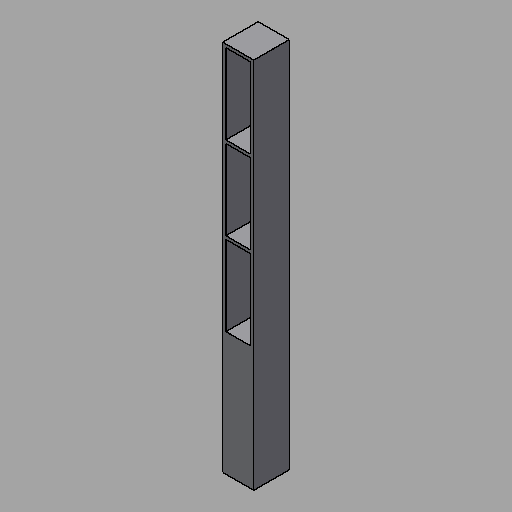
# Autodesk Inventor part: Mobiletto verticale
Saved by Autodesk Inventor 2025.2 (Build 292293000, 293)
## iProperties
Created: 2025-09-19
Part Number: Mobiletto verticale
Material: Generico
Document SubType Name: Modeling
Designer: Limonta
Mass: 39347.7 g
Surface Area: 22881.9 cm^2
Volume: 39347.7 cm^3
Density: 1 g/cm^3
Appearance: Default
FORNITO DA: SBE
Author: Limonta
Autodesk Inventor part; units mm, degrees
ref_plane "YZ Plane" through (0, 0, 0) normal (1, 0, 0) x (0, 1, 0)
ref_plane "XZ Plane" through (0, 0, 0) normal (0, 1, 0) x (-1, 0, 0)
ref_plane "XY Plane" through (0, 0, 0) normal (0, 0, 1) x (1, 0, 0)
sketch "Schizzo1" plane through (0, 0, 0) normal (0, 0, 1) x (1, 0, 0)
  line L0 (-87.5, 0) -> (87.5, 0)
  line L1 (87.5, 0) -> (87.5, 2100)
  line L2 (87.5, 2100) -> (-87.5, 2100)
  line L3 (-87.5, 2100) -> (-87.5, 0)
  point P0 (0, 0)
  point P1 (0, 0)
  dimension "d0" = 175
  dimension "d1" = 2100
  constraints: 8 end point, 2 parallel, 1 coincident, 1 horizontal, 1 midpoint, 1 perpendicular
  measures "d0" distance of L0.start L0.end
  measures "d1" distance of L2.end L0.start
extrude "Estrusione1" add sketch "Schizzo1" against normal blind 200
shell "Svuotamento1" thickness 18 removed faces 1 at (-29.1667, 1400, 0)
sketch "Schizzo2" plane through (0, 0, 0) normal (0, 0, 1) x (1, 0, 0)
  line L0 (-69.5, 18) -> (-69.5, 2082) projected
  line L1 (69.5, 2082) -> (69.5, 18) projected
  line L2 (-69.5, 1632) -> (69.5, 1632)
  line L3 (69.5, 1632) -> (69.5, 1614)
  line L4 (69.5, 1614) -> (-69.5, 1614)
  line L5 (-69.5, 1614) -> (-69.5, 1632)
  line L6 (-69.5, 1164) -> (69.5, 1164)
  line L7 (69.5, 1164) -> (69.5, 1146)
  line L8 (69.5, 1146) -> (-69.5, 1146)
  line L9 (-69.5, 1146) -> (-69.5, 1164)
  line L10 (-69.5, 18) -> (-69.5, 2082) projected
  line L11 (69.5, 2082) -> (69.5, 18) projected
  line L12 (-69.5, 696) -> (69.5, 696)
  line L13 (69.5, 696) -> (69.5, 18)
  line L14 (69.5, 18) -> (-69.5, 18)
  line L15 (-69.5, 18) -> (-69.5, 696)
  point P0 (0, 0)
  point P1 (69.5, 1614)
  point P2 (69.5, 1632)
  point P3 (-69.5, 1632)
  point P4 (69.5, 1146)
  point P5 (69.5, 1164)
  point P6 (-69.5, 1164)
  point P7 (69.5, 18)
  dimension "d6" = 18
  dimension "d7" = 450
  dimension "d8" = 450
  dimension "d12" = 450
  dimension "d13" = 678
  constraints: 24 end point, 6 parallel, 4 collinear, 3 horizontal, 3 perpendicular, 3 point on line
  measures "d6" distance between parallel lines of L4 L2
  measures "d7" distance from line of L2 L0.end
  measures "d8" distance between parallel lines of L6 L4
  measures "d12" distance between parallel lines of L12 L8
  measures "d13" distance of L0.start L12.start
extrude "Estrusione2" add sketch "Schizzo2" against normal up to surface (182 mm away) contours L0 L12 L1 L14 | L0 L6 L1 L8 | L0 L2 L1 L4
equation "\"d8\" = d7"
equation "\"d12\" = d7"
